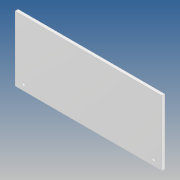
# Autodesk Inventor part: KB33-046-004-014 - Лицевая вертикальня пластина
Saved by Autodesk Inventor 2020 (Build 240168000, 168)
## iProperties
Created: 2021-06-26
Part Number: KB33-046-004-014 - Лицевая вертикальня пластина
Material: Пластик АБС
Document SubType Name: Modeling
Designer: Петров Иван
Mass: 77.3586 g
Surface Area: 389.344 cm^2
Volume: 72.9798 cm^3
Density: 1.06 g/cm^3
Appearance: Гладкий — белый
Author: Петров Иван
Autodesk Inventor part; units mm, degrees
ref_plane "YZ Plane" through (0, 0, 0) normal (1, 0, 0) x (0, 1, 0)
ref_plane "XZ Plane" through (0, 0, 0) normal (0, 1, 0) x (-1, 0, 0)
ref_plane "XY Plane" through (0, 0, 0) normal (0, 0, 1) x (1, 0, 0)
sketch "Эскиз1" plane through (0, 0, 0) normal (0, 0, 1) x (1, 0, 0)
  line L0 (-26.3955, 0) -> (-26.3955, 30) projected
  line L1 (168.6045, 0) -> (168.6045, 30) projected
  circle A0 centre (161.1045, 7.5) radius 2 projected
  circle A1 centre (-18.8955, 7.5) radius 2 projected
  line L2 (-26.3955, 60.0004) -> (-30.3955, 60.0004) projected
  line L3 (172.6045, 60.0004) -> (168.6045, 60.0004) projected
  line L4 (-26.3955, 60.0004) -> (168.6045, 60.0004)
  line L5 (168.6045, 60.0004) -> (168.6045, 0)
  line L6 (168.6045, 0) -> (-26.3955, 0)
  line L7 (-26.3955, 0) -> (-26.3955, 60.0004)
  point P0 (0, 0)
  constraints: 8 end point, 2 parallel, 1 horizontal, 1 perpendicular
extrude "Выдавливание1" add sketch "Эскиз1" along normal blind 4
thicken "Толщина1" operation add thickness 4 both sides no extend neighbours yes toward (1, 0, 0) faces at (168.6045, 10, 1.3333) (168.6045, 40.0001, 2.6667)
thicken "Толщина2" operation add thickness 4 both sides no extend neighbours yes toward (-1, 0, 0) faces at (-26.3955, 40.0003, 2.6667)
sketch "Эскиз2" plane through (0, 0, 4) normal (0, 0, 1) x (1, 0, 0)
  line L0 (172.6045, 60.0004) -> (-30.3955, 60.0004) projected
  line L1 (-30.3955, 60.0004) -> (172.6045, 60.0004)
  line L2 (172.6045, 60.0004) -> (172.6045, 90.0004)
  line L3 (172.6045, 90.0004) -> (-30.3955, 90.0004)
  line L4 (-30.3955, 90.0004) -> (-30.3955, 60.0004)
  point P0 (0, 0)
  dimension "d6" = 30
  constraints: 8 end point, 2 parallel, 1 horizontal, 1 perpendicular
  measures "d6" distance of L2.end L1.end
extrude "Выдавливание2" add sketch "Эскиз2" against normal blind 4
